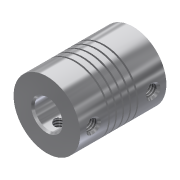
# Autodesk Inventor part: shaft couple_flex
Saved by Autodesk Inventor 2014 (Build 180170000, 170)
## iProperties
Created: 2015-11-28
Part Number: shaft couple_flex
Material: Generic
Document SubType Name: Modeling
Designer: Tom
Density: 1 g/cm^3
Appearance: Default
Author: Tom
Autodesk Inventor part; units mm, degrees
ref_plane "YZ Plane" through (0, 0, 0) normal (1, 0, 0) x (0, 1, 0)
ref_plane "XY Plane" through (0, 0, 0) normal (0, 0, 1) x (1, 0, 0)
sketch "Sketch1" plane through (0, 0, 0) normal (0, 0, 1) x (1, 0, 0)
  circle A0 centre (0, 0) radius 9.525
  circle A1 centre (0, 0) radius 2.5
  dimension "d0" = 19.05
  dimension "d1" = 5
  constraints: 2 centre point, 2 coincident
  measures "d0" diameter of A0
  measures "d1" diameter of A1
extrude "Extrusion1" add sketch "Sketch1" along normal blind 24.638
sketch "Sketch3" plane through (0, 0, 24.638) normal (0, 0, 1) x (1, 0, 0)
  circle A0 centre (0, 0) radius 2.5 projected
  circle A1 centre (0, 0) radius 2.5 projected
  circle A2 centre (0, 0) radius 4
  dimension "d4" = 8
  constraints: 1 centre point, 1 coincident
  measures "d4" diameter of A2
extrude "Extrusion2" cut sketch "Sketch3" against normal blind 17.526
sketch "Sketch5" plane through (0, 0, 0) normal (0, 1, 0) x (-1, 0, 0)
  line L0 (4, 24.638) -> (4, 7.112) projected
  line L1 (4, 17.1704) -> (9.9129, 17.1704)
  line L2 (9.9129, 17.1704) -> (9.9129, 17.6022)
  line L3 (9.9129, 17.6022) -> (4, 17.6022)
  line L4 (4, 17.6022) -> (4, 17.1704)
  line L5 (0, 0) -> (0, -7.0667)
  line L6 (-9.525, 0) -> (9.525, 0) projected
  line L7 (9.525, 24.638) -> (-9.525, 24.638) projected
  dimension "d8" = 0.4318
  dimension "d17" = 7.0358
  constraints: 10 end point, 2 parallel, 2 perpendicular, 1 horizontal, 1 point on line
  measures "d8" distance from line of L3 L1.end
  measures "d17" distance from line of L7 L2.end
coil "Coil1" sketch "Sketch5" operation cut axis through (0, 0, 0) along (0, 0, -1) pitch 2.032 turns 5 hand right
sketch "Sketch6" plane through (0, 0, 0) normal (0, 1, 0) x (-1, 0, 0)
  circle A0 centre (0, 20.828) radius 2
  line L0 (9.525, 24.638) -> (-9.525, 24.638) projected
  line L1 (2.5, 0) -> (-2.5, 0) projected
  circle A1 centre (0, 3.81) radius 2
  point P0 (0, 0)
  dimension "d18" = 4
  dimension "d19" = 3.81
  dimension "d20" = 4
  dimension "d21" = 3.81
  constraints: 2 centre point
  measures "d18" diameter of A0
  measures "d19" distance from line of L0 A0.centre
  measures "d20" diameter of A1
  measures "d21" distance of point (0, 0) A1.centre
hole "Hole1" at (0, 0, 20.828) at (0, 0, 3.81) direction (0, -1, 0) diameter 3.2512 end through all
ref_plane "Work Plane2" through (0, 0, 24.638) normal (1, 0, 0) x (0, 0, -1)
sketch "Sketch8" plane through (0, 0, 24.638) normal (1, 0, 0) x (0, 0, -1)
  circle A0 centre (20.8388, 0) radius 2
  circle A1 centre (3.81, 0) radius 2
  line L0 (0, -4) -> (0, 4) projected
  point P0 (24.638, 0)
  dimension "d30" = 4
  dimension "d31" = 4
  dimension "d32" = 3.81
  dimension "d33" = 3.7992
  constraints: 2 centre point
  measures "d30" diameter of A0
  measures "d31" diameter of A1
  measures "d32" distance from line of A1.centre L0
  measures "d33" distance of point (24.638, 0) A0.centre
hole "Hole2" at (0, 0, 20.828) at (0, 0, 3.7992) direction (1, 0, 0) diameter 3.2512 end through all
chamfer "Chamfer1" distance 0.5 angle 45 6 edges at (-2.5, 0, 0) (-4, 0, 24.638) (9.3853, 1.6256, 20.8278) (9.3853, -1.6256, 20.8282) (9.3853, -1.6256, 3.7994) (9.3853, 1.6256, 3.799)
chamfer "Chamfer2" distance 0.5 angle 45 2 edges at (-0.5541, -9.5089, 2.2818) (-0.5541, -9.5089, 19.2998)
body "Solid1"
